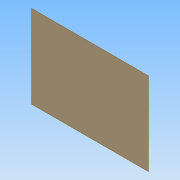
# Autodesk Inventor part: A4-paper
Saved by Autodesk Inventor 2016 (Build 200138000, 138)
## iProperties
Created: 2015-10-22
Part Number: A4-paper
Material: Generic
Document SubType Name: Modeling
Designer: Openlab
Density: 1 g/cm^3
Appearance: Smooth - Off-White
Author: Openlab
Autodesk Inventor part; units mm, degrees
ref_plane "YZ Plane" through (0, 0, 0) normal (1, 0, 0) x (0, 1, 0)
ref_plane "XZ Plane" through (0, 0, 0) normal (0, 1, 0) x (-1, 0, 0)
ref_plane "XY Plane" through (0, 0, 0) normal (0, 0, 1) x (1, 0, 0)
sketch "Sketch1" plane through (0, 0, 0) normal (0, 1, 0) x (-1, 0, 0)
  line L0 (103.1524, 141.4823) -> (-193.8476, 141.4823)
  line L1 (-193.8476, 141.4823) -> (-193.8476, -68.5177)
  line L2 (-193.8476, -68.5177) -> (103.1524, -68.5177)
  line L3 (103.1524, -68.5177) -> (103.1524, 141.4823)
  point P0 (0, 0)
  dimension "d0" = 210
  dimension "d1" = 297
  constraints: 8 end point, 2 parallel, 1 horizontal, 1 perpendicular
  measures "d0" distance of L2.end L0.start
  measures "d1" distance of L0.start L0.end
extrude "Extrusion1" add sketch "Sketch1" along normal blind 0.2
body "Solid1"
